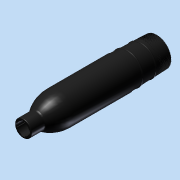
# Autodesk Inventor part: Body_Sleeve
Saved by Autodesk Inventor 2012 (Build 160160000, 160)
## iProperties
Created: 2015-03-22
Part Number: Body_Sleeve
Material: Default
Document SubType Name: Modeling
Designer: Jason
Density: 1 g/cm^3
Author: Jason
Autodesk Inventor part; units mm, degrees
ref_plane "XZ Plane" through (0, 0, 0) normal (0, 1, 0) x (-1, 0, 0)
ref_plane "XY Plane" through (0, 0, 0) normal (0, 0, 1) x (1, 0, 0)
sketch "Sketch2" plane through (0, 0, 0) normal (1, 0, 0) x (0, 1, 0)
  line L0 (0, 0) -> (0, 32.25)
  line L1 (0, 0) -> (5.4, 0)
  line L2 (5.4, 0) -> (5.4, 20.25)
  line L3 (5.4, 20.25) -> (0, 20.25) construction
  line L4 (0, 32.25) -> (2.8, 32.25)
  line L5 (2.8, 32.25) -> (2.8, 27.65)
  arc A0 (5.4, 20.25) -> (2.8, 27.65) centre (-6.4308, 20.25) ccw
  line L6 (0, -6.45) -> (0, 38.7) projected
  dimension "d0" = 5.4
  dimension "d1" = 12
  dimension "d2" = 4.6
  dimension "d3" = 2.8
  dimension "d4" = 32.25
  constraints: 12 end point, 3 horizontal, 3 vertical, 2 point on circle, 1 centre point, 1 point on line, 1 tangent
  measures "d0" distance between parallel lines of L0 L2
  measures "d1" distance between parallel lines of L4 L3
  measures "d2" distance of L4.end L5.end
  measures "d3" distance of L0.end L4.end
  measures "d4" distance between parallel lines of L1 L4
revolve "Revolution1" add sketch "Sketch2" angle 360 about axis through (0, 0, -10) along (0, 0, 1)
fillet "Fillet1" radius 1 1 edges at (0, -2.8, 27.65)
shell "Shell1" thickness 0.75 removed faces 1 at (0.8727, -0.331, 32.25)
sketch "Sketch4" plane through (0, 0, 32.25) normal (0, 0, 1) x (1, 0, 0)
  circle A0 centre (0, 0) radius 2.05 construction
  circle A1 centre (0, 0) radius 2.8 construction
  arc A2 (0.6, 2.2204) -> (-0.6, 2.2204) centre (0, 0) ccw
  line L0 (-0.6, 1.3748) -> (-0.6, 2.2204)
  line L1 (0.6, 1.3748) -> (0.6, 2.2204)
  arc A3 (0.6, 1.3748) -> (-0.6, 1.3748) centre (0, 0) ccw
  point P0 (0, 2.3)
  point P1 (0, 1.5)
  dimension "d11" = 0.5
  dimension "d12" = 1.2
  dimension "d13" = 1.5
  constraints: 6 point on circle, 4 end point, 2 centre point, 2 coincident, 2 vertical, 2 vertical alignment
  measures "d11" radial gap between concentric circles of A1 A2
  measures "d12" distance between parallel lines of L1 L0
  measures "d13" radius of A3
extrude "Extrusion2" cut sketch "Sketch4" against normal blind 10
pattern_circular "Circular Pattern1" count 4 over 360 about axis through (0, 0, -10) along (0, 0, 1) of "Extrusion2"
fillet "Fillet2" radius 0.2 1 edges at (0, -2.8, 32.25)
sketch "Sketch7" plane through (0, 0, 0.75) normal (0, 0, 1) x (1, 0, 0)
  circle A0 centre (0, 0) radius 4.65 projected
extrude "Hole" cut sketch "Sketch7" against normal blind 10
sketch "Sketch8" plane through (0, 0, 0) normal (1, 0, 0) x (0, 1, 0)
  line L0 (-5.3, 0) -> (-4.8, -12.88) construction
  line L1 (-4.8, -12.88) -> (-3.8993, -12.88) construction
  line L2 (-3.8993, -12.88) -> (-4.3993, 0)
  line L3 (-5.3, 0) -> (-4.3993, 0)
  line L4 (4.65, 0) -> (-4.65, 0) projected
  line L5 (0, -21.906) -> (0, 41.276) projected
  line L6 (-4.75, -12.88) -> (-4.8663, -9.8823)
  line L7 (-4.8663, -9.8823) -> (-4.9164, -9.8823)
  line L8 (-4.75, -12.88) -> (-3.8993, -12.88)
  line L9 (-4.9164, -9.8823) -> (-5.3, 0)
  point P0 (0, 0)
  point P1 (-4.8497, 0)
  dimension "d23" = 5.3
  dimension "d24" = 12.88
  dimension "d25" = 0.9
  dimension "d26" = 4.8
  dimension "d28" = 3
  dimension "d29" = 0.05
  constraints: 16 end point, 4 horizontal, 3 parallel, 2 point on line, 1 horizontal alignment, 1 midpoint
  measures "d23" distance of L0.start point (0, 0)
  measures "d24" distance between parallel lines of L1 L4
  measures "d25" distance between parallel lines of L0 L2
  measures "d26" horizontal distance of point (0, 0) L0.end
  measures "d28" distance of L6.start L6.end
  measures "d29" distance between parallel lines of L0 L6
revolve "Revolution2" add sketch "Sketch8" angle 360 about axis through (0, 0, -10) along (0, 0, 1)
ref_plane "Work Plane1" through (-6, 0, 0) normal (1, 0, 0) x (0, 1, 0)
sketch "Sketch11" plane through (0, 0, 0) normal (1, 0, 0) x (0, 1, 0)
  line L0 (-5.3, 0) -> (-4.8, -12.88) construction
  line L1 (-5.0053, -8.88) -> (-4.85, -12.88)
  line L2 (-4.9052, -8.88) -> (-4.75, -12.88)
  line L3 (-4.85, -12.88) -> (-4.75, -12.88)
  line L4 (-4.8, -12.88) -> (-3.8993, -12.88) construction
  line L5 (-5.0053, -8.88) -> (-4.9052, -8.88)
  point P0 (0, 0)
  dimension "d35" = 0.1
  dimension "d36" = 0.05
  dimension "d37" = 4
  constraints: 8 end point, 2 horizontal, 1 collinear
  measures "d35" distance between parallel lines of L1 L2
  measures "d36" distance between parallel lines of L0 L1
  measures "d37" distance between parallel lines of L4 L5
extrude "Fix" add sketch "Sketch11" along normal mid plane 0.1
pattern_circular "Circular Pattern2" count 90 over 360 about axis through (0, 0, -10) along (0, 0, 1) of "Fix"
sketch "Sketch13" plane through (0, 0, 0) normal (1, 0, 0) x (0, 1, 0)
  line L0 (-5.3, 0) -> (-4.8, -12.88) construction
  arc A0 (-5.1979, -2.63) -> (-5.1746, -3.23) centre (-5.061, -2.9251) ccw
  line L1 (-5.1979, -2.63) -> (-5.1746, -3.23)
  line L2 (5.3, 0) -> (-5.3, 0) construction
  line L3 (0, -21.906) -> (0, 41.276) projected
  line L4 (-5.3864, -2.5998) -> (-5.061, -2.5998) construction
  line L5 (-5.061, -2.5998) -> (-5.061, -3.2505) construction
  line L6 (-5.061, -3.2505) -> (-5.3864, -3.2505) construction
  line L7 (-5.3864, -3.2505) -> (-5.3864, -2.5998) construction
  point P0 (0, 0)
  dimension "d43" = 0.6
  dimension "d44" = 0.2
  dimension "d45" = 2.63
  constraints: 10 end point, 3 tangent, 2 parallel, 2 point on circle, 2 point on line, 1 centre point, 1 coincident, 1 collinear, 1 horizontal, 1 midpoint, 1 perpendicular
  measures "d43" vertical distance of L1.end L1.start
  measures "d44" distance edge to line of A0 L0
  measures "d45" distance from line of L2 L1.start
revolve "Revolution3" add sketch "Sketch13" angle 360 about axis through (0, 0, -10) along (0, 0, 1)
sketch "Sketch14" plane through (0, 0, 0) normal (1, 0, 0) x (0, 1, 0)
  line L0 (-5.3, 0) -> (-4.8, -12.88) construction
  arc A0 (-5.0174, -7.2807) -> (-4.9941, -7.8807) centre (-4.8805, -7.5758) ccw
  line L1 (-4.9941, -7.8807) -> (-5.0174, -7.2807)
  line L2 (-5.2058, -7.2505) -> (-4.6168, -7.2505) construction
  line L3 (-4.6168, -7.2505) -> (-4.6168, -7.9012) construction
  line L4 (-4.6168, -7.9012) -> (-5.2058, -7.9012) construction
  line L5 (-5.2058, -7.9012) -> (-5.2058, -7.2505) construction
  line L6 (-5.061, -3.2505) -> (-5.3864, -3.2505) construction
  line L7 (0, -21.906) -> (0, 41.276) projected
  point P0 (0, 0)
  dimension "d50" = 0.2
  dimension "d51" = 0.6
  dimension "d52" = 4
  constraints: 10 end point, 3 tangent, 2 parallel, 2 point on circle, 2 point on line, 1 centre point, 1 collinear, 1 horizontal, 1 perpendicular
  measures "d50" distance edge to line of A0 L0
  measures "d51" vertical distance of L1.start L1.end
  measures "d52" distance between parallel lines of L2 L6
revolve "Revolution4" add sketch "Sketch14" angle 360 about axis through (0, 0, -10) along (0, 0, 1)
chamfer "Chamfer1" distance 0.6 distance2 1 1 edges at (0, 3.8993, -12.88) measured on face at (-2.3665, -3.426, -12.88)
equation "\"d36\" = 0.5 * d35"
equation "\"d50\" = d44"
equation "\"d51\" = d43"
body "Solid1"
